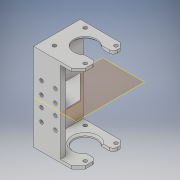
# Autodesk Inventor part: mount
Saved by Autodesk Inventor 2019 (Build 230136000, 136)
## iProperties
Created: 2020-04-12
Part Number: mount
Material: Generisch
Document SubType Name: Modeling
Designer: marc
Density: 1 g/cm^3
Appearance: Vorgabe
Author: marc
## iProperties of the stored document mount_3D-Druck.ipt
Created: 2020-06-20
Part Number: mount_3D-Druck
Material: Generisch
Document SubType Name: Modeling
Designer: marc
Density: 1 g/cm^3
Appearance: Vorgabe
Author: marc
Autodesk Inventor part; units mm, degrees
ref_plane "YZ Plane" through (0, 0, 0) normal (1, 0, 0) x (0, 1, 0)
ref_plane "XZ Plane" through (0, 0, 0) normal (0, 1, 0) x (-1, 0, 0)
ref_plane "XY Plane" through (0, 0, 0) normal (0, 0, 1) x (1, 0, 0)
sketch "Skizze1" plane through (0, 0, 0) normal (0, 1, 0) x (-1, 0, 0)
  line L0 (0, 0) -> (42, 0)
  line L1 (42, 0) -> (42, 42)
  line L2 (42, 42) -> (0, 42)
  line L3 (0, 42) -> (0, 0)
  dimension "d0" = 42
  dimension "d1" = 42
  constraints: 8 end point, 2 parallel, 1 horizontal, 1 perpendicular
  measures "d0" distance of L2.end L1.end
  measures "d1" distance of L1.end L0.end
extrude "Extrusion1" add sketch "Skizze1" along normal blind 3
sketch "Skizze2" plane through (0, 3, 0) normal (0, 1, 0) x (1, 0, 0)
  line L0 (-42, 0) -> (-42, -42) projected
  line L1 (-42, -42) -> (0, -42) projected
  point P0 (0, 0)
  point P1 (-35, -33)
  point P2 (-35, -2)
  point P3 (-4, -2)
  point P4 (-4, -33)
  dimension "d4" = 31
  dimension "d5" = 31
  dimension "d6" = 7
  dimension "d7" = 9
  dimension "d8" = 42
  constraints: 2 horizontal alignment, 2 vertical alignment
  measures "d4" distance of point (-35, -2) point (-35, -33)
  measures "d5" distance of point (-4, -33) point (-35, -33)
  measures "d6" distance from line of L0 point (-35, -33)
  measures "d7" distance from line of L1 point (-35, -33)
  measures "d8" distance of L0.end L1.end
hole "Bohrung1" at (-35, 3, 2) at (-4, 3, 2) at (-4, 3, 33) at (-35, 3, 33) direction (0, -1, 0) diameter 3.6 end through all clearance for "Flachkopfsenkschraube DIN EN ISO 2009" size "M3" standard "DIN"
ref_plane "Arbeitsebene1" through (0, 44, 0) normal (0, 1, 0) x (1, 0, 0)
mirror "Spiegeln1" about plane through (0, 44, 0) normal (0, 1, 0)
sketch "Skizze4" plane through (-42, 0, 0) normal (-1, 0, 0) x (0, 0, 1)
  line L0 (0, 88) -> (42, 88) projected
  line L1 (42, 88) -> (0, 88)
  line L2 (0, 88) -> (0, 0)
  line L3 (0, 0) -> (42, 0)
  line L4 (42, 0) -> (42, 88)
  constraints: 8 end point, 2 parallel, 1 horizontal, 1 perpendicular
extrude "Extrusion2" add sketch "Skizze4" along normal blind 3
sketch "Skizze5" plane through (0, 0, 0) normal (0, -1, 0) x (1, 0, 0)
  circle A0 centre (-4, 33) radius 1.8 projected
  point P0 (0, 0)
  point P1 (-19.5, 17.5)
  dimension "d19" = 15.5
  dimension "d20" = 15.5
  measures "d19" horizontal distance of A0.centre point (-19.5, 17.5)
  measures "d20" horizontal distance of A0.centre point (-19.5, 17.5)
hole "Bohrung2" at (-19.5, 0, 17.5) direction (0, 1, 0) diameter 23 end through all
sketch "Skizze6" plane through (-42, 0, 0) normal (1, 0, 0) x (0, 0, -1)
  line L0 (-42, 85) -> (0, 85) projected
  line L1 (0, 3) -> (-42, 3) projected
  line L2 (-42, 85) -> (-39, 85)
  line L3 (-39, 85) -> (-39, 3)
  line L4 (-39, 3) -> (-42, 3)
  line L5 (-42, 3) -> (-42, 85)
  point P0 (0, 0)
  dimension "d28" = 3
  constraints: 8 end point, 2 parallel, 1 horizontal, 1 perpendicular, 1 point on line
  measures "d28" distance of L3.end L4.end
extrude "Extrusion3" add sketch "Skizze6" along normal blind 24
sketch "Skizze7" plane through (0, 44, 0) normal (0, 1, 0) x (1, 0, 0)
  line L0 (-18, -39) -> (-42, -39)
  line L1 (-42, -39) -> (-42, 0)
  line L2 (-42, 0) -> (-18, 0)
  line L3 (-18, 0) -> (-18, -39)
  point P0 (0, 0)
  point P1 (-42, -39)
  constraints: 8 end point, 2 parallel, 1 horizontal, 1 perpendicular
extrude "Extrusion4" add sketch "Skizze7" along normal mid plane 1
chamfer "Fase1" distance 24 angle 45 1 edges at (-18, 44, 0)
sketch "Skizze8" plane through (-18, 85, 39) normal (0, 0, -1) x (-1, 0, 0)
  line L0 (0, -40.5) -> (0, 0) projected
  line L1 (24, -40.5) -> (0, -40.5) projected
  line L2 (-18, 0) -> (24, 0) projected
  line L3 (24, -40.5) -> (24, 0) projected
  point P0 (-18, -85)
  point P1 (5, -35.5)
  point P2 (5, -23)
  point P3 (19, -23)
  point P4 (19, -35.5)
  dimension "d36" = 5
  dimension "d37" = 5
  dimension "d39" = 5
  dimension "d92" = 12.5
  constraints: 2 horizontal alignment, 2 vertical alignment
  measures "d36" distance from line of L0 point (5, -35.5)
  measures "d37" distance from line of L1 point (5, -35.5)
  measures "d39" distance from line of L3 point (19, -23)
  measures "d92" distance of point (5, -35.5) point (5, -23)
hole "Bohrung3" at (-23, 49.5, 39) at (-23, 62, 39) at (-37, 62, 39) at (-37, 49.5, 39) direction (0, 0, 1) diameter 3.6 end through all clearance for "Flachkopfsenkschraube DIN EN ISO 2009" size "M3" standard "DIN"
sketch "Skizze9" plane through (-18, 85, 39) normal (0, 0, -1) x (-1, 0, 0)
  line L0 (1.7668, -35.5) -> (3.3834, -32.7)
  line L1 (3.3834, -32.7) -> (6.6166, -32.7)
  line L2 (6.6166, -32.7) -> (8.2332, -35.5)
  line L3 (8.2332, -35.5) -> (6.6166, -38.3)
  line L4 (6.6166, -38.3) -> (3.3834, -38.3)
  line L5 (3.3834, -38.3) -> (1.7668, -35.5)
  line L6 (1.7668, -23) -> (3.3834, -20.2)
  line L7 (3.3834, -20.2) -> (6.6166, -20.2)
  line L8 (6.6166, -20.2) -> (8.2332, -23)
  line L9 (8.2332, -23) -> (6.6166, -25.8)
  line L10 (6.6166, -25.8) -> (3.3834, -25.8)
  line L11 (3.3834, -25.8) -> (1.7668, -23)
  line L12 (15.45, -35.5) -> (17.225, -32.4256)
  line L13 (17.225, -32.4256) -> (20.775, -32.4256)
  line L14 (20.775, -32.4256) -> (22.55, -35.5)
  line L15 (22.55, -35.5) -> (20.775, -38.5744)
  line L16 (20.775, -38.5744) -> (17.225, -38.5744)
  line L17 (17.225, -38.5744) -> (15.45, -35.5)
  line L18 (15.7668, -23) -> (17.3834, -20.2)
  line L19 (17.3834, -20.2) -> (20.6166, -20.2)
  line L20 (20.6166, -20.2) -> (22.2332, -23)
  line L21 (22.2332, -23) -> (20.6166, -25.8)
  line L22 (20.6166, -25.8) -> (17.3834, -25.8)
  line L23 (17.3834, -25.8) -> (15.7668, -23)
  circle A0 centre (5, -35.5) radius 1.8 projected
  circle A1 centre (5, -23) radius 1.8 projected
  circle A2 centre (19, -35.5) radius 1.8 projected
  circle A3 centre (19, -23) radius 1.8 projected
  line L24 (-18, 0) -> (24, 0) projected
  point P0 (-18, -85)
  dimension "d47" = 5.6
  dimension "d48" = 5.6
  constraints: 48 end point, 4 coincident, 4 parallel, 1 horizontal alignment, 1 point on line, 52 other
  measures "d47" distance between parallel lines of L4 L1
  measures "d48" distance between parallel lines of L7 L10
extrude "Extrusion5" cut sketch "Skizze9" against normal blind 2.5
mirror "Spiegeln2" about plane through (0, 44, 0) normal (0, 1, 0) of "Extrusion5", "Bohrung3"
move faces "Verschieben1" translate (0, 0, -3) faces at (-44, 43.8333, 0)
chamfer "Fase2" distance 5 angle 45 4 edges at (0, 86.5, -3) (0, 1.5, -3) (0, 1.5, 42) (0, 86.5, 42)
chamfer "Fase3" distance 1.75 angle 45 2 edges at (-19.5, 3, 29) (-19.5, 85, 29)
sketch "Skizze10" plane through (-45, 88, 42) normal (0, 1, 0) x (1, 0, 0)
  line L0 (45, 5) -> (45, 40) projected
  line L1 (33, 16) -> (45, 16)
  line L2 (45, 16) -> (45, 33)
  line L3 (45, 33) -> (33, 33)
  line L4 (33, 33) -> (33, 16)
  line L5 (40, 45) -> (0, 45) projected
  line L6 (0, 0) -> (40, 0) projected
  point P0 (45, 42)
  dimension "d60" = 12
  dimension "d61" = 16
  dimension "d62" = 12
  constraints: 8 end point, 2 parallel, 1 horizontal, 1 perpendicular, 1 point on line
  measures "d60" distance from line of L5 L3.end
  measures "d61" distance between parallel lines of L6 L1
  measures "d62" distance between parallel lines of L0 L4
extrude "Extrusion6" cut sketch "Skizze10" against normal up to surface (88 mm away)
fillet "Rundung1" radius 4 4 edges at (0, 1.5, 9) (0, 1.5, 26) (0, 86.5, 26) (0, 86.5, 9)
move faces "Verschieben2" translate (0, 0, 2) faces at (-33.1897, 78.9159, 42)
sketch "Skizze11" plane through (0, 0, 0) normal (0, -1, 0) x (1, 0, 0)
  line L0 (-45, -3) -> (-33.2803, -23.299)
  line L1 (-33.2803, -23.299) -> (-31.0303, -22)
  line L2 (-5, -3) -> (-42, -3) projected
  line L3 (-31.0303, -22) -> (-42, -3)
  line L4 (-5, -3) -> (-45, -3) projected
  point P0 (0, 0)
  dimension "d69" = 90
  dimension "d70" = 19
  dimension "d71" = 3
  dimension "d72" = 60
  constraints: 6 end point, 1 perpendicular, 1 point on line
  measures "d69" angle of L0 L1
  measures "d70" distance from line of L2 L1.end
  measures "d71" distance of L0.start L2.end
  measures "d72" angle of L0 L4
extrude "Extrusion7" [suppressed]
sketch "Skizze12" plane through (-19.5, 88, 17.5) normal (0, 1, 0) x (1, 0, 0)
  line L0 (-11.5303, 39.5) -> (-22.5, 20.5) projected
  line L1 (-16.5, 30.8923) -> (-16.5, 20.5)
  line L2 (14.5, 20.5) -> (-25.5, 20.5) projected
  point P0 (19.5, 17.5)
  dimension "d75" = 90
  dimension "d76" = 6
  constraints: 2 end point, 2 point on line
  measures "d75" angle of L2 L1
  measures "d76" distance of L0.end L1.end
extrude "Extrusion8" [suppressed]
mirror "Spiegeln3" [suppressed]
sketch "Skizze13" plane through (-33.2803, 0, -23.299) normal (-0.8660254, 0, -0.5) x (-0.5, 0, 0.8660254)
  line L0 (3, 1) -> (11, 1)
  line L1 (11, 1) -> (11, 18)
  line L2 (11, 18) -> (3, 18)
  line L3 (3, 18) -> (3, 1)
  circle A0 centre (7, 22) radius 1.7
  line L4 (0, 0) -> (0, 52) projected
  line L5 (23.4393, 0) -> (0, 0) projected
  point P0 (3.5374, 0)
  dimension "d79" = 4
  dimension "d80" = 17
  dimension "d81" = 8
  dimension "d82" = 4
  dimension "d83" = 3.4
  dimension "d84" = 3
  dimension "d85" = 1
  constraints: 8 end point, 2 parallel, 1 centre point, 1 horizontal, 1 perpendicular
  measures "d79" distance from line of L2 A0.centre
  measures "d80" distance of L2.end L0.start
  measures "d81" distance of L0.start L0.end
  measures "d82" distance from line of L3 A0.centre
  measures "d83" diameter of A0
  measures "d84" distance between parallel lines of L4 L3
  measures "d85" distance between parallel lines of L5 L0
extrude "Extrusion9" [suppressed]
mirror "Spiegeln4" [suppressed]
sketch "Skizze14" plane through (0, 44, 0) normal (0, 1, 0) x (1, 0, 0)
  line L0 (-36.5303, 12.4737) -> (-42, 3) projected
  line L1 (-42, 3) -> (-36.5303, 12.4737) projected
  line L2 (-36.5303, 12.4737) -> (-32.5303, 19.4019) projected
  line L3 (-32.5303, 19.4019) -> (-36, 13.3923) projected
  line L4 (-31.0303, 22) -> (-36, 13.3923) projected
  line L5 (-31.0303, 22) -> (-36, 13.3923) projected
  line L6 (-36, 13.3923) -> (-32.5303, 19.4019) projected
  line L7 (-32.5303, 19.4019) -> (-36.5303, 12.4737) projected
  line L8 (-33.6803, 17.4101) -> (-35.3803, 14.4656) projected
  line L9 (-33.6803, 17.4101) -> (-35.3803, 14.4656) projected
  line L10 (-42, 0) -> (-18, -24) projected
  line L11 (-18, -24) -> (-42, 0) projected
  line L12 (-36, 13.3923) -> (-32.3987, -9.6013)
  line L13 (-42, 0) -> (-18, -24) projected
  line L14 (-42, 3) -> (-42, -39) projected
  line L15 (-42, -39) -> (-42, 0) projected
  line L16 (-42, 0) -> (-42, -39) projected
  line L17 (-42, 3) -> (-42, -39) projected
  line L18 (-42, 0) -> (-32.3987, -9.6013)
  line L19 (-18, -24) -> (-42, 0) projected
  line L20 (-42, 0) -> (-42.3696, 2.3598)
  line L21 (-42.3696, 2.3598) -> (-36, 13.3923)
  point P0 (0, 0)
  dimension "d89" = 8
  constraints: 8 end point, 2 collinear, 2 point on line, 1 parallel
  measures "d89" distance between parallel lines of L12 L20
extrude "Extrusion10" [suppressed]
equation "\"d20\" = d19"
equation "\"d48\" = d47"
equation "\"d82\" = 0.5 * d81"
